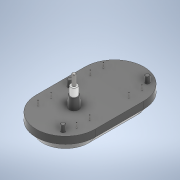
# Autodesk Inventor part: BKA
Saved by Autodesk Inventor 2020 (Build 240168000, 168)
## iProperties
Created: 2019-07-03
Part Number: BKA
Material: ABS Plastic
Document SubType Name: Modeling
Designer: andwh
Density: 1.06 g/cm^3
Appearance: Smooth - Black
Author: andwh
Autodesk Inventor part; units mm, degrees
ref_plane "YZ Plane" through (0, 0, 0) normal (1, 0, 0) x (0, 1, 0)
ref_plane "XZ Plane" through (0, 0, 0) normal (0, 1, 0) x (-1, 0, 0)
ref_plane "XY Plane" through (0, 0, 0) normal (0, 0, 1) x (1, 0, 0)
sketch "Sketch1" plane through (0, 0, 0) normal (0, 1, 0) x (-1, 0, 0)
  circle A0 centre (-11.43, -21.12) radius 0.25
  circle A1 centre (-11.43, -28.88) radius 0.25
  circle A2 centre (-9, -34.5) radius 1.25
  line L0 (11.43, -28.88) -> (-11.43, -28.88) construction
  circle A3 centre (11.43, -21.12) radius 0.25
  circle A4 centre (11.43, -28.88) radius 0.25
  arc A5 (-17.5, -24) -> (17.5, -24) centre (0, -24) ccw
  circle A6 centre (11.43, 2.12) radius 0.25
  circle A7 centre (-11.43, 9.88) radius 0.25
  circle A8 centre (11.43, 9.88) radius 0.25
  circle A9 centre (-9, 15.5) radius 1.25
  arc A10 (17.5, 5) -> (-17.5, 5) centre (0, 5) ccw
  circle A11 centre (-11.43, 2.12) radius 0.25
  circle A12 centre (12, -9.5) radius 1.25
  line L1 (17.5, -24) -> (17.5, 5)
  line L2 (11.43, -21.12) -> (11.43, 2.12) construction
  line L3 (0, -24) -> (0, 5) construction
  line L4 (-17.5, 5) -> (-17.5, -24)
  line L5 (-9, -34.5) -> (-9, 15.5) construction
  circle A13 centre (0, 0) radius 2.75
  point P0 (0, -41.5)
  point P1 (0, -28.88)
  point P2 (0, 22.5)
  point P3 (-9, -9.5)
  point P4 (11.43, -9.5)
  point P5 (0, -9.5)
  dimension "d0" = 17.5
  dimension "d2" = 5.5
  dimension "d3" = 64
  dimension "d4" = 2.5
  dimension "d5" = 12
  dimension "d6" = 50
  dimension "d7" = 9
  dimension "d8" = 22.86
  dimension "d9" = 7.76
  dimension "d10" = 7.76
  dimension "d11" = 23.24
  dimension "d12" = 0.5
  dimension "d13" = 9.5
  constraints: 14 centre point, 14 end point, 12 coincident, 9 equal radius, 7 vertical alignment, 6 horizontal alignment, 6 point on circle, 4 midpoint, 4 tangent, 3 vertical, 1 horizontal, 1 parallel, 1 point on line
  measures "d0" radius of A5
  measures "d2" diameter of A13
  measures "d3" distance of point (0, 22.5) point (0, -41.5)
  measures "d4" diameter of A12
  measures "d5" distance from line of L3 A12.centre
  measures "d6" distance of L5.start L5.end
  measures "d7" distance between parallel lines of L3 L5
  measures "d8" distance of L0.start L0.end
  measures "d9" distance of L2.start L0.start
  measures "d10" distance of point (11.43, 9.88) L2.end
  measures "d11" distance of L2.start L2.end
  measures "d12" diameter of A4
  measures "d13" distance of point (0, 0) point (0, -9.5)
extrude "Extrusion1" add sketch "Sketch1" against normal blind 9.2 contours A0 | A1 | A2 | A3 | A4 | L4 A10 L1 A5 | A6 | A7 | A8 | A9 | A11 | A12 | A13
chamfer "Chamfer1" distance 4 distance2 5 4 edges at (0, -9.2, 22.5) (-17.5, -9.2, -9.5) (0, -9.2, -41.5) (17.5, -9.2, -9.5) measured on face at (17, -9.2, -9.5) measured on face at (0, -9.2, -41) measured on face at (0, -9.2, 22) measured on face at (-17, -9.2, -9.5)
extrude "Extrusion2" add sketch "Sketch1" along normal blind 2.8 contours A0 | A1 | A3 | A4 | A6 | A7 | A8 | A11
extrude "Extrusion3" add sketch "Sketch1" along normal blind 3.8 contours A2 | A9 | A12
chamfer "Chamfer2" distance 0.2 angle 45 3 edges at (-10.75, 3.8, -9.5) (10.25, 3.8, 15.5) (10.25, 3.8, -34.5)
extrude "Extrusion4" add sketch "Sketch1" along normal blind 6.4 contours A13
chamfer "Chamfer3" distance 0.25 distance2 6.4 1 edges at (2.75, 6.4, 0) measured on face at (2.25, 6.4, 0)
sketch "Sketch3" plane through (0, 6.4, 0) normal (0, 1, 0) x (1, 0, 0)
  circle A0 centre (0, 0) radius 2
  dimension "d31" = 4
  constraints: 1 centre point, 1 coincident
  measures "d31" diameter of A0
extrude "Extrusion5" add sketch "Sketch3" along normal blind 4.8
sketch "Sketch4" plane through (0, 11.2, 0) normal (0, 1, 0) x (1, 0, 0)
  circle A0 centre (0, 0) radius 1
  dimension "d34" = 2
  constraints: 1 centre point, 1 coincident
  measures "d34" diameter of A0
extrude "Extrusion6" add sketch "Sketch4" along normal blind 6.2
chamfer "Chamfer4" distance 0.25 angle 45 1 edges at (-1, 17.4, 0)
equation "\"d10\" = d9"
body "Solid1"
